Autodesk Fusion 360 part; units mm, degrees
(part 2 of 2)
  spline S123 degree 3 poles (-3.5792, -37.4673) (-3.5789, -37.47) (-3.5787, -37.4727) (-3.5784, -37.4754) (-3.5616, -37.6538) (-3.5457, -37.8429) (-3.468, -38.0189) (-3.3909, -38.1936) (-3.2631, -38.3322) (-3.1438, -38.4642) (-3.1413, -38.467) (-3.1388, -38.4697) (-3.1363, -38.4725) knots -0.000796 -0.000796 -0.000796 -0.000796 0 0 0 0.052256 0.052256 0.052256 0.104169 0.104169 0.104169 0.105252 0.105252 0.105252 0.105252
  spline S124 degree 3 poles (-3.1363, -38.4725) (-3.1333, -38.4746) (-3.1302, -38.4767) (-3.1272, -38.4789) (-2.9735, -38.5872) (-2.8134, -38.7015) (-2.6264, -38.7699) (-2.4165, -38.8466) (-2.1951, -38.8572) (-1.9836, -38.8687) (-1.982, -38.8688) (-1.9803, -38.8689) (-1.9786, -38.869) knots -0.001092 -0.001092 -0.001092 -0.001092 0 0 0 0.055294 0.055294 0.055294 0.117384 0.117384 0.117384 0.117873 0.117873 0.117873 0.117873
  spline S125 degree 3 poles (-1.9786, -38.869) (-1.977, -38.8689) (-1.9753, -38.8689) (-1.9736, -38.8688) (-1.7608, -38.8592) (-1.5378, -38.8507) (-1.3264, -38.7733) (-1.1458, -38.7071) (-0.9912, -38.5969) (-0.8429, -38.4926) (-0.8393, -38.49) (-0.8356, -38.4875) (-0.832, -38.4849) knots -0.000488 -0.000488 -0.000488 -0.000488 0 0 0 0.062379 0.062379 0.062379 0.115684 0.115684 0.115684 0.116993 0.116993 0.116993 0.116993
  spline S126 degree 3 poles (-0.832, -38.4849) (-0.8291, -38.4815) (-0.8263, -38.478) (-0.8234, -38.4746) (-0.7121, -38.3403) (-0.5933, -38.1996) (-0.5216, -38.0271) (-0.4431, -37.8383) (-0.4315, -37.6365) (-0.4186, -37.4455) (-0.4185, -37.4431) (-0.4183, -37.4406) (-0.4182, -37.4382) knots -0.001303 -0.001303 -0.001303 -0.001303 0 0 0 0.051012 0.051012 0.051012 0.106831 0.106831 0.106831 0.107534 0.107534 0.107534 0.107534
  spline S127 degree 3 poles (-0.4182, -37.4382) (-0.4183, -37.4358) (-0.4185, -37.4334) (-0.4187, -37.431) (-0.4288, -37.3008) (-0.4389, -37.1678) (-0.4606, -37.0339) (-0.482, -36.902) (-0.5138, -36.7739) (-0.5479, -36.6483) knots -0.000721 -0.000721 -0.000721 -0.000721 0 0 0 0.039096 0.039096 0.039096 0.077625 0.077625 0.077625 0.077625
  line L52 (1.1891, -36.7736) -> (-0.5479, -36.6483)
  spline S128 degree 3 poles (1.1891, -36.7736) (1.1847, -36.8084) (1.1807, -36.8437) (1.1776, -36.8795) (1.173, -36.934) (1.1709, -36.9873) (1.1688, -37.0391) (1.1688, -37.041) (1.1687, -37.043) (1.1686, -37.0449) knots 0.010573 0.010573 0.010573 0.010573 0.020792 0.020792 0.020792 0.036334 0.036334 0.036334 0.036916 0.036916 0.036916 0.036916
  spline S129 degree 3 poles (1.1686, -37.0449) (1.1688, -37.0468) (1.1689, -37.0488) (1.169, -37.0507) (1.1822, -37.2237) (1.1946, -37.4065) (1.2626, -37.5801) (1.3278, -37.7463) (1.4361, -37.8838) (1.5376, -38.015) (1.5395, -38.0174) (1.5414, -38.0199) (1.5433, -38.0224) knots -0.000568 -0.000568 -0.000568 -0.000568 0 0 0 0.050801 0.050801 0.050801 0.09941 0.09941 0.09941 0.100327 0.100327 0.100327 0.100327
  spline S130 degree 3 poles (1.5433, -38.0224) (1.5456, -38.0244) (1.548, -38.0265) (1.5503, -38.0286) (1.6704, -38.135) (1.7971, -38.2497) (1.9571, -38.3192) (2.1123, -38.3866) (2.277, -38.402) (2.4316, -38.4182) (2.4344, -38.4184) (2.4372, -38.4187) (2.44, -38.419) knots -0.000913 -0.000913 -0.000913 -0.000913 0 0 0 0.046854 0.046854 0.046854 0.092288 0.092288 0.092288 0.093106 0.093106 0.093106 0.093106
  spline S131 degree 3 poles (2.44, -38.419) (2.4428, -38.4188) (2.4456, -38.4187) (2.4484, -38.4185) (2.5906, -38.4094) (2.7433, -38.4015) (2.8898, -38.3434) (3.0231, -38.2907) (3.1315, -38.2042) (3.2334, -38.1247) (3.2368, -38.1221) (3.2401, -38.1194) (3.2435, -38.1168) knots -0.000817 -0.000817 -0.000817 -0.000817 0 0 0 0.04166 0.04166 0.04166 0.079551 0.079551 0.079551 0.0808 0.0808 0.0808 0.0808
  spline S132 degree 3 poles (3.2435, -38.1168) (3.2461, -38.1134) (3.2487, -38.1101) (3.2513, -38.1067) (3.3308, -38.0029) (3.417, -37.8928) (3.4697, -37.7583) (3.529, -37.6068) (3.5362, -37.4487) (3.5446, -37.3012) (3.5447, -37.2991) (3.5448, -37.2971) (3.5449, -37.295) knots -0.00125 -0.00125 -0.00125 -0.00125 0 0 0 0.038322 0.038322 0.038322 0.081498 0.081498 0.081498 0.082102 0.082102 0.082102 0.082102
  spline S133 degree 3 poles (3.5449, -37.295) (3.5448, -37.2929) (3.5447, -37.2909) (3.5445, -37.2888) (3.5342, -37.135) (3.5249, -36.971) (3.4637, -36.8141) (3.4072, -36.669) (3.3139, -36.5496) (3.2274, -36.4366) (3.2245, -36.4328) (3.2215, -36.4289) (3.2186, -36.425) knots -0.000605 -0.000605 -0.000605 -0.000605 0 0 0 0.045123 0.045123 0.045123 0.086852 0.086852 0.086852 0.088276 0.088276 0.088276 0.088276
  spline S134 degree 3 poles (3.2186, -36.425) (3.2146, -36.4222) (3.2107, -36.4193) (3.2068, -36.4165) (3.0749, -36.3207) (2.9381, -36.2205) (2.7811, -36.1489) (2.6017, -36.0671) (2.411, -36.0297) (2.2242, -35.9988) knots -0.001438 -0.001438 -0.001438 -0.001438 0 0 0 0.048282 0.048282 0.048282 0.103467 0.103467 0.103467 0.103467
  line L53 (2.6565, -33.5863) -> (2.2242, -35.9988)
  spline S135 degree 3 poles (2.6565, -33.5863) (3.0079, -33.7032) (3.3472, -33.8257) (3.6311, -34.0165) (3.9209, -34.2111) (4.1681, -34.4872) (4.4192, -34.771) knots 0.011325 0.011325 0.011325 0.011325 0.120727 0.120727 0.120727 0.232387 0.232387 0.232387 0.232387
  spline S136 degree 3 poles (4.4192, -34.771) (4.6117, -35.1348) (4.7997, -35.4934) (4.9073, -35.866) (5.0414, -36.3302) (5.0565, -36.8362) (5.0705, -37.3507) knots 0.00118 0.00118 0.00118 0.00118 0.123135 0.123135 0.123135 0.275027 0.275027 0.275027 0.275027
  spline S137 degree 3 poles (5.0705, -37.3507) (5.0621, -37.9271) (5.0522, -38.4938) (4.8926, -39.0069) (4.7743, -39.3869) (4.5699, -39.7506) (4.3605, -40.1195) knots 0.000205 0.000205 0.000205 0.000205 0.169641 0.169641 0.169641 0.295126 0.295126 0.295126 0.295126
  spline S138 degree 3 poles (4.3605, -40.1195) (4.1066, -40.3707) (3.8584, -40.6115) (3.5744, -40.7453) (3.2939, -40.8774) (2.9545, -40.9164) (2.6039, -40.9537) knots 0.001338 0.001338 0.001338 0.001338 0.105226 0.105226 0.105226 0.207833 0.207833 0.207833 0.207833
  spline S139 degree 3 poles (2.6039, -40.9537) (2.3966, -40.9394) (2.1969, -40.9243) (2.0175, -40.8697) (1.8401, -40.8157) (1.6675, -40.7185) (1.4891, -40.6165) knots 0.000862 0.000862 0.000862 0.000862 0.062366 0.062366 0.062366 0.123203 0.123203 0.123203 0.123203
  spline S140 degree 3 poles (1.4891, -40.6165) (1.3178, -40.4779) (1.1513, -40.3421) (1.0144, -40.1878) (0.8562, -40.0096) (0.7282, -39.7962) (0.5975, -39.5771) (0.5565, -39.5085) (0.5156, -39.4399) (0.4746, -39.3713) knots 0.000799 0.000799 0.000799 0.000799 0.066407 0.066407 0.066407 0.14223 0.14223 0.14223 0.16598 0.16598 0.16598 0.16598
  spline S141 degree 3 poles (0.4746, -39.3713) (0.4547, -39.4487) (0.4347, -39.526) (0.4148, -39.6034) (0.3701, -39.7767) (0.3262, -39.9458) (0.2635, -40.1029) (0.2156, -40.2232) (0.1545, -40.3418) (0.0917, -40.4632) knots -0.023875 -0.023875 -0.023875 -0.023875 0 0 0 0.053461 0.053461 0.053461 0.094361 0.094361 0.094361 0.094361
  spline S142 degree 3 poles (0.0917, -40.4632) (-0.0169, -40.6177) (-0.1226, -40.7663) (-0.2473, -40.8854) (-0.3703, -41.0028) (-0.5215, -41.1007) (-0.6785, -41.2011) knots 0.000666 0.000666 0.000666 0.000666 0.056767 0.056767 0.056767 0.112153 0.112153 0.112153 0.112153
  spline S143 degree 3 poles (-0.6785, -41.2011) (-0.8567, -41.2805) (-1.0299, -41.3567) (-1.2047, -41.3994) (-1.3991, -41.4469) (-1.6096, -41.4566) (-1.8267, -41.4655) knots 0.000741 0.000741 0.000741 0.000741 0.05877 0.05877 0.05877 0.123308 0.123308 0.123308 0.123308
  spline S144 degree 3 poles (-1.8267, -41.4655) (-2.1147, -41.4455) (-2.3963, -41.425) (-2.6574, -41.3548) (-2.9258, -41.2826) (-3.1863, -41.1543) (-3.4522, -41.022) knots 0.000546 0.000546 0.000546 0.000546 0.086282 0.086282 0.086282 0.174445 0.174445 0.174445 0.174445
  spline S145 degree 3 poles (-3.4522, -41.022) (-3.7029, -40.8526) (-3.9469, -40.6862) (-4.1394, -40.4823) (-4.3361, -40.2741) (-4.4903, -40.0148) (-4.647, -39.7485) knots 0.000656 0.000656 0.000656 0.000656 0.090235 0.090235 0.090235 0.181711 0.181711 0.181711 0.181711
  spline S146 degree 3 poles (-2.0504, -47.0996) (-2.051, -47.0989) (-2.0516, -47.0983) (-2.0521, -47.0976) (-2.1404, -46.9941) (-2.2293, -46.8898) (-2.3218, -46.7876) (-2.4337, -46.664) (-2.5491, -46.5454) (-2.6637, -46.4277) (-2.7209, -46.3689) (-2.7781, -46.31) (-2.8353, -46.2512) knots -0.000262 -0.000262 -0.000262 -0.000262 0 0 0 0.040795 0.040795 0.040795 0.090071 0.090071 0.090071 0.114681 0.114681 0.114681 0.114681
  line L54 (-2.8353, -50.7357) -> (-2.8353, -46.2512)
  line L55 (-4.9, -50.7357) -> (-2.8353, -50.7357)
  line L56 (-4.9, -42.6199) -> (-4.9, -50.7357)
  spline S147 degree 3 poles (-4.9, -42.6199) (-4.5327, -42.6868) (-4.1722, -42.7586) (-3.8368, -42.883) (-3.4578, -43.0235) (-3.0987, -43.2357) (-2.735, -43.4519) knots 0.011882 0.011882 0.011882 0.011882 0.123237 0.123237 0.123237 0.249052 0.249052 0.249052 0.249052
  spline S148 degree 3 poles (-2.735, -43.4519) (-2.3289, -43.7861) (-1.9256, -44.1185) (-1.5623, -44.4848) (-1.0597, -44.9915) (-0.6257, -45.5712) (-0.1892, -46.1548) knots 0.00076 0.00076 0.00076 0.00076 0.158042 0.158042 0.158042 0.375637 0.375637 0.375637 0.375637
  spline S149 degree 3 poles (-0.1892, -46.1549) (0.0642, -46.4996) (0.3198, -46.8477) (0.6159, -47.1643) (0.8027, -47.3639) (1.0028, -47.5481) (1.201, -47.7306) (1.2029, -47.7323) (1.2048, -47.7341) (1.2067, -47.7358) knots 0.000083 0.000083 0.000083 0.000083 0.128023 0.128023 0.128023 0.208705 0.208705 0.208705 0.209469 0.209469 0.209469 0.209469
  spline S150 degree 3 poles (1.2067, -47.7358) (1.2088, -47.7372) (1.2109, -47.7386) (1.213, -47.74) (1.3608, -47.8393) (1.5149, -47.9442) (1.6944, -48.0072) (1.8457, -48.0603) (2.0014, -48.0789) (2.15, -48.0973) (2.1537, -48.0978) (2.1574, -48.0982) (2.161, -48.0987) knots -0.000753 -0.000753 -0.000753 -0.000753 0 0 0 0.052523 0.052523 0.052523 0.096837 0.096837 0.096837 0.097933 0.097933 0.097933 0.097933
  spline S151 degree 3 poles (2.161, -48.0987) (2.1647, -48.0983) (2.1684, -48.098) (2.1721, -48.0976) (2.3193, -48.0832) (2.4766, -48.0695) (2.6255, -48.0056) (2.7765, -47.9408) (2.896, -47.8343) (3.0091, -47.7358) (3.0115, -47.7337) (3.014, -47.7316) (3.0164, -47.7294) knots -0.001083 -0.001083 -0.001083 -0.001083 0 0 0 0.04321 0.04321 0.04321 0.087001 0.087001 0.087001 0.087951 0.087951 0.087951 0.087951
  spline S152 degree 3 poles (3.0164, -47.7294) (3.0184, -47.7269) (3.0204, -47.7243) (3.0224, -47.7217) (3.1169, -47.5999) (3.2183, -47.4716) (3.2795, -47.3159) (3.3438, -47.1522) (3.355, -46.9805) (3.3671, -46.8186) (3.3673, -46.8162) (3.3675, -46.8138) (3.3677, -46.8113) knots -0.000953 -0.000953 -0.000953 -0.000953 0 0 0 0.045202 0.045202 0.045202 0.092709 0.092709 0.092709 0.093426 0.093426 0.093426 0.093426
  spline S153 degree 3 poles (3.3677, -46.8113) (3.3675, -46.8089) (3.3673, -46.8064) (3.3671, -46.804) (3.3551, -46.6367) (3.344, -46.4591) (3.2767, -46.2906) (3.2136, -46.1326) (3.1091, -46.0028) (3.0116, -45.8795) (3.0086, -45.8757) (3.0056, -45.8719) (3.0026, -45.868) knots -0.000716 -0.000716 -0.000716 -0.000716 0 0 0 0.049062 0.049062 0.049062 0.09511 0.09511 0.09511 0.096531 0.096531 0.096531 0.096531
  spline S154 degree 3 poles (3.0026, -45.868) (2.9986, -45.8653) (2.9946, -45.8625) (2.9907, -45.8597) (2.8412, -45.7546) (2.6868, -45.6452) (2.5114, -45.5678) (2.302, -45.4753) (2.0789, -45.4359) (1.8603, -45.4027) knots -0.001438 -0.001438 -0.001438 -0.001438 0 0 0 0.054151 0.054151 0.054151 0.118802 0.118802 0.118802 0.118802
  line L57 (2.0691, -42.8207) -> (1.8603, -45.4027)
  spline S155 degree 3 poles (2.0691, -42.8207) (2.3873, -42.8723) (2.699, -42.9284) (2.9894, -43.031) (3.2489, -43.1226) (3.5, -43.2545) (3.755, -43.3892) knots 0.010744 0.010744 0.010744 0.010744 0.106995 0.106995 0.106995 0.19299 0.19299 0.19299 0.19299
  spline S156 degree 3 poles (3.755, -43.3892) (3.9605, -43.5509) (4.1598, -43.7094) (4.3143, -43.8951) (4.4773, -44.0909) (4.6009, -44.3293) (4.7266, -44.5748) knots 0.000893 0.000893 0.000893 0.000893 0.078417 0.078417 0.078417 0.160124 0.160124 0.160124 0.160124
  spline S157 degree 3 poles (4.7266, -44.5748) (4.8278, -44.8855) (4.9271, -45.1923) (4.9844, -45.5018) (5.058, -45.8997) (5.0645, -46.3152) (5.0705, -46.7363) knots 0.000789 0.000789 0.000789 0.000789 0.098326 0.098326 0.098326 0.22376 0.22376 0.22376 0.22376
  spline S158 degree 3 poles (5.0705, -46.7363) (5.0653, -47.174) (5.0597, -47.6065) (4.9884, -48.023) (4.9337, -48.3427) (4.8391, -48.6602) (4.7428, -48.9814) knots 0.00013 0.00013 0.00013 0.00013 0.130639 0.130639 0.130639 0.230794 0.230794 0.230794 0.230794
  spline S159 degree 3 poles (4.7428, -48.9814) (4.6194, -49.2349) (4.498, -49.4811) (4.3347, -49.6832) (4.176, -49.8798) (3.968, -50.0468) (3.7535, -50.2172) knots 0.0008 0.0008 0.0008 0.0008 0.084251 0.084251 0.084251 0.165384 0.165384 0.165384 0.165384
  spline S160 degree 3 poles (3.7535, -50.2172) (3.517, -50.3522) (3.2862, -50.4822) (3.0465, -50.555) (2.803, -50.629) (2.5345, -50.6486) (2.2584, -50.6673) knots 0.000756 0.000756 0.000756 0.000756 0.081349 0.081349 0.081349 0.163224 0.163224 0.163224 0.163224
  spline S161 degree 3 poles (2.2584, -50.6673) (1.9569, -50.6433) (1.6625, -50.6187) (1.393, -50.5379) (1.112, -50.4536) (0.8427, -50.3036) (0.5677, -50.1489) knots 0.000726 0.000726 0.000726 0.000726 0.090356 0.090356 0.090356 0.18381 0.18381 0.18381 0.18381
  spline S162 degree 3 poles (0.5677, -50.1489) (0.2679, -49.9095) (-0.0285, -49.6722) (-0.2904, -49.4072) (-0.6393, -49.054) (-0.9357, -48.6428) (-1.2347, -48.227) knots 0.000804 0.000804 0.000804 0.000804 0.115403 0.115403 0.115403 0.268105 0.268105 0.268105 0.268105
  spline S163 degree 3 poles (-1.2347, -48.227) (-1.3964, -47.9922) (-1.5587, -47.7565) (-1.7288, -47.5253) (-1.834, -47.3822) (-1.9416, -47.2417) (-2.0488, -47.1017) (-2.0494, -47.101) (-2.0499, -47.1003) (-2.0504, -47.0996) knots 0.000103 0.000103 0.000103 0.000103 0.085612 0.085612 0.085612 0.138511 0.138511 0.138511 0.138774 0.138774 0.138774 0.138774
  dimension "d168" = 0.1
  dimension "d169" = 0.1
  dimension "d170" = 0.1
  dimension "d171" = 0.1
  dimension "d172" = 0.1
extrude "Extrude1'''''" add sketch "Sketch1 (7)" along normal blind 1 separate body contours L29 L30 L31 L32 L33 L34 L35 L36 L37 L38 L39 L40 | S82 S83 S84 S85 S86 L41 S87 S88 S89 S90 S91 S92 S93 S94 S95 S96 S97 S98 S99 L42 S100 S101 S102 S103 S104 S105 S106 S107 S108 | L43 S109 S110 S111 S112 L44 L45 L46 L47 | S117 S118 S119 S120 L51 S121 S122 S123 S124 S125 S126 S127 L52 S128 S129 S130 S131 S132 S133 S134 L53 S135 S136 S137 S138 S139 S140 S141 S142 S143 S144 S145 | S146 L54 L55 L56 S147 S148 S149 S150 S151 S152 S153 S154 L57 S155 S156 S157 S158 S159 S160 S161 S162 S163 makes body 6 at (-0.2122, 24.8027, 6.5) makes body 7 at (-0.2081, 19.4836, 6.5) makes body 8 at (-0.4359, 38.3237, 6.5) makes body 9 at (0.2213, 4.6299, 6.5) makes body 10 at (4.2118, 46.5356, 6.5) in component "Letters"
component "Board" placed x (1, 0, 0) y (0, 1, 0) z (0, 0, 1) at (0, 0, 0)
component "Bottom" placed x (1, 0, 0) y (0, 1, 0) z (0, 0, 1) at (0, 0, 0)
component "Top" placed x (1, 0, 0) y (0, 1, 0) z (0, 0, 1) at (0, 0, 0)
component "Latch" placed x (1, 0, 0) y (0, 1, 0) z (0, 0, 1) at (15.75, 13.6, 0)
component "Light Pipe" placed x (1, 0, 0) y (0, 1, 0) z (0, 0, 1) at (0, 0, 0)
component "Letters" placed x (1, 0, 0) y (0, 1, 0) z (0, 0, 1) at (0, 0, 0)
equation "board_width = 27.9 mm"
equation "board_length = 54.4 mm"
equation "d3 = board_width"
equation "d4 = board_length"
equation "module_height = 3.4 mm"
equation "usb_height = 2.7 mm"
equation "led_height = 0.7 mm"
equation "pcb_thickness = 1.6 mm"
equation "d18 = -pcb_thickness"
equation "d20 = module_height"
equation "d22 = led_height"
equation "d24 = usb_height"
equation "tolerance_small = 0.1 mm"
equation "tolerance_big = 0.3 mm"
equation "wall_thickness_sides = 3 mm"
equation "wall_thickness_top_and_bottom = 1 mm"
equation "d32 = board_width + 2 * tolerance_big"
equation "d33 = board_length + 2 * tolerance_big"
equation "d34 = tolerance_big"
equation "d35 = -wall_thickness_sides"
equation "box_bottom_height = 9 mm" comment "not less than 9"
equation "d37 = -box_bottom_height"
equation "d39 = -box_bottom_height + wall_thickness_top_and_bottom"
equation "box_top_height = 7 mm" comment "not less than 7"
equation "d42 = box_top_height"
equation "d44 = box_top_height - wall_thickness_top_and_bottom"
equation "d46 = -tolerance_small"
equation "d48 = -wall_thickness_sides"
equation "d50 = -wall_thickness_sides"
equation "d52 = -wall_thickness_sides + 0.8 mm"
equation "d54 = -wall_thickness_sides + 0.8 mm"
equation "d58 = board_length / 2"
equation "d59 = -box_bottom_height + pcb_thickness + tolerance_small"
equation "d66 = board_length - 15 mm"
equation "d67 = -box_top_height + module_height + tolerance_small"
equation "d69 = -box_top_height + usb_height + tolerance_small"
equation "d71 = -wall_thickness_sides / 2 + tolerance_small"
equation "d72 = -wall_thickness_sides / 2 - tolerance_small"
equation "rim_height = 2 mm"
equation "d74 = -rim_height"
equation "d76 = -rim_height"
equation "latch_bottom_width = 7 mm"
equation "latch_top_width = 10 mm"
equation "latch_lock_distance = 8 mm"
equation "d81 = latch_bottom_width / 2"
equation "d82 = latch_top_width / 2"
equation "filament_diameter = 1.75 mm"
equation "latch_hole_diameter = filament_diameter + 2 * tolerance_big"
equation "d85 = latch_lock_distance / 2"
equation "d86 = latch_hole_diameter / 2"
equation "d87 = latch_hole_diameter + 2 mm"
equation "d90 = latch_lock_distance / 2"
equation "latch_thickness = 1 mm"
equation "d93 = latch_thickness / 2"
equation "latch_count_on_side = 2"
equation "latch_y = ( board_length / latch_count_on_side ) / 2"
equation "latch_x = board_width / 2 + tolerance_big + wall_thickness_sides / 2"
equation "d100 = latch_y"
equation "d101 = latch_x"
equation "d107 = latch_thickness + 2 * tolerance_big"
equation "d108 = latch_bottom_width + 2 * tolerance_big"
equation "d109 = latch_lock_distance / 2 + latch_hole_diameter / 2 + 1 mm + tolerance_big"
equation "d111 = rim_height"
equation "d113 = latch_hole_diameter"
equation "d114 = latch_lock_distance / 2"
equation "d115 = -wall_thickness_sides / 2"
equation "d118 = latch_count_on_side"
equation "d120 = -board_length / latch_count_on_side"
equation "d123 = latch_thickness + 2 * tolerance_big"
equation "d124 = latch_bottom_width + 2 * tolerance_big"
equation "d125 = latch_thickness + 2 * tolerance_big"
equation "d126 = latch_top_width + 2 mm"
equation "d127 = latch_x"
equation "d128 = latch_y"
equation "d129 = -box_bottom_height"
equation "d131 = -box_bottom_height + latch_lock_distance / 2 - 2 * tolerance_small"
equation "d134 = latch_count_on_side"
equation "d135 = latch_x * 2"
equation "d136 = -( board_length / latch_count_on_side )"
equation "d139 = board_length / 2"
equation "d140 = rim_height"
equation "d141 = wall_thickness_sides / 2"
equation "d143 = filament_diameter + 4 * tolerance_small"
equation "d145 = -wall_thickness_top_and_bottom"
equation "d147 = -box_top_height + led_height + tolerance_big"
equation "d149 = filament_diameter"
equation "d150 = -box_top_height + led_height + tolerance_big"
equation "d163 = board_length"
equation "d164 = board_width"
equation "d167 = -tolerance_small"
equation "d168 = tolerance_small"
equation "d169 = tolerance_small"
equation "d170 = tolerance_small"
equation "d171 = tolerance_small"
equation "d172 = tolerance_small"
